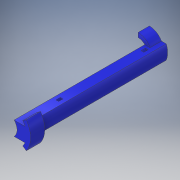
# Autodesk Inventor part: insert
Saved by Autodesk Inventor 2017 (Build 210142000, 142)
## iProperties
Created: 2018-12-03
Part Number: insert
Material: Generic
Document SubType Name: Modeling
Designer: ddeboer
Density: 1 g/cm^3
Appearance: Default
Author: ddeboer
Autodesk Inventor part; units mm, degrees
ref_plane "YZ Plane" through (0, 0, 0) normal (1, 0, 0) x (0, 1, 0)
ref_plane "XZ Plane" through (0, 0, 0) normal (0, 1, 0) x (-1, 0, 0)
ref_plane "XY Plane" through (0, 0, 0) normal (0, 0, 1) x (1, 0, 0)
sketch "Sketch1" plane through (0, 0, 0) normal (0, 0, 1) x (1, 0, 0)
  arc A0 (13.516, -9.464) -> (13.516, 9.464) centre (0, 0) ccw
  arc A1 (11.0586, -7.7433) -> (11.0586, 7.7433) centre (0, 0) ccw
  line L0 (11.0586, 7.7433) -> (13.516, 9.464)
  line L1 (0, 0) -> (16.5, 0) construction
  line L2 (11.0586, -7.7433) -> (13.516, -9.464)
  line L3 (0, 0) -> (16.5, 0) construction
  dimension "d0" = 33
  dimension "d1" = 27
  dimension "d2" = 35
  dimension "d3" = 35
  constraints: 8 end point, 4 point on circle, 2 centre point, 2 coincident, 2 horizontal
  measures "d0" diameter of A0
  measures "d1" diameter of A1
  measures "d2" angle of L1 L0
  measures "d3" angle of L2 L3
extrude "Extrusion1" add sketch "Sketch1" along normal blind 10
sketch "Sketch2" plane through (0, 0, 10) normal (0, 0, 1) x (1, 0, 0)
  line L0 (4.6804, -5.0196) -> (14.6804, -5.0196)
  line L1 (14.6804, -5.0196) -> (14.6804, 4.9804)
  line L2 (14.6804, 4.9804) -> (4.6804, 4.9804)
  line L3 (4.6804, 4.9804) -> (4.6804, -5.0196)
  line L4 (4.6804, -0.0196) -> (14.6804, -0.0196) construction
  point P0 (0, 0)
  dimension "d6" = 10
  dimension "d7" = 10
  constraints: 10 end point, 2 midpoint, 2 parallel, 1 horizontal, 1 perpendicular
  measures "d6" distance of L2.end L1.end
  measures "d7" distance of L1.end L0.end
extrude "Extrusion2" add sketch "Sketch2" against normal blind 100
sketch "Sketch4" plane through (0, 0, 0) normal (0, 0, -1) x (-1, 0, 0)
  circle A0 centre (0, 0) radius 18.2384
  circle A1 centre (0, 0) radius 13
  dimension "d14" = 26
  constraints: 2 centre point, 2 coincident
  measures "d14" diameter of A1
extrude "Extrusion4" cut sketch "Sketch4" along normal blind 100
sketch "Sketch5" plane through (0, 0, 10) normal (0, 0, 1) x (1, 0, 0)
  circle A0 centre (0, 0) radius 7
  dimension "d17" = 14
  constraints: 1 centre point, 1 coincident
  measures "d17" diameter of A0
extrude "Extrusion5" cut sketch "Sketch5" against normal blind 100
sketch "Sketch9" plane through (11.0586, 7.7433, 10) normal (-0.5735764, 0.819152, 0) x (0.819152, 0.5735764, 0)
  line L0 (-3.014, 87) -> (-4.614, 87)
  line L1 (-4.614, 87) -> (-4.614, 90)
  line L2 (-4.614, 90) -> (-3.014, 90)
  line L3 (-3.014, 90) -> (-3.014, 87)
  line L4 (-6.614, 100) -> (-0.8069, 100) projected
  line L5 (-6.614, 100) -> (-6.614, 0) projected
  line L6 (-13.5, 120) -> (-13.5, -20) projected
  point P0 (-13.5, 10)
  dimension "d34" = 1.6
  dimension "d35" = 3
  dimension "d36" = 10
  dimension "d37" = 2
  constraints: 8 end point, 2 parallel, 1 horizontal, 1 perpendicular
  measures "d34" distance of L1.end L2.end
  measures "d35" distance of L0.end L1.end
  measures "d36" distance between parallel lines of L2 L4
  measures "d37" distance between parallel lines of L1 L5
revolve "Revolution4" cut sketch "Sketch9" angle 360 about axis through (0, 0, -10) along (0, 0, 1)
pattern_linear "Rectangular Pattern2" count 2 spacing 60 along (0, 0, 1) of "Revolution4"
ref_plane "Work Plane1" through (13.516, -9.464, 0) normal (-0.5735764, -0.819152, 0) x (0.819152, -0.5735764, 0)
sketch "Sketch10" plane through (13.516, -9.464, 0) normal (-0.5735764, -0.819152, 0) x (0.819152, -0.5735764, 0)
  line L0 (-15.3273, -90) -> (-9.5202, -90) projected
  line L1 (-9.5202, -90) -> (-6.5202, -90)
  line L2 (-6.5202, -90) -> (-6.5202, -82)
  line L3 (-6.5202, -82) -> (-9.5202, -82)
  line L4 (-9.5202, -82) -> (-9.5202, -90)
  line L5 (-16.5, -110) -> (-16.5, 30) projected
  point P0 (-16.5, 0)
  dimension "d43" = 3
  dimension "d44" = 8
  constraints: 8 end point, 2 parallel, 1 horizontal, 1 perpendicular
  measures "d43" distance of L3.end L2.end
  measures "d44" distance of L2.end L1.end
revolve "Revolution5" add sketch "Sketch10" angle 360 about axis through (0, 0, -10) along (0, 0, 1)
sketch "Sketch11" plane through (4.8789, -5.0196, -82) normal (0, 0, 1) x (1, 0, 0)
  line L0 (-4.7394, -7.0475) -> (-15.4812, -7.0475)
  line L1 (-15.4812, -7.0475) -> (-15.4812, 15.7614)
  line L2 (-15.4812, 15.7614) -> (-4.7394, 15.7614)
  line L3 (-4.7394, 15.7614) -> (-4.7394, -7.0475)
  point P0 (-4.8789, 5.0196)
  constraints: 8 end point, 2 parallel, 1 horizontal, 1 perpendicular
extrude "Extrusion7" cut sketch "Sketch11" along normal mid plane 200
body "Solid1"
